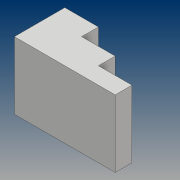
# Autodesk Inventor part: 46 (44000.000 mm^3)
Saved by Autodesk Inventor 2018 (Build 220112000, 112)
## iProperties
Created: 2020-09-18
Part Number: 46 (44000.000 mm^3)
Material: 一般
Document SubType Name: Modeling
Designer: 88697
Density: 1 g/cm^3
Appearance: 預設
Author: 88697
Autodesk Inventor part; units mm, degrees
ref_plane "YZ Plane" through (0, 0, 0) normal (1, 0, 0) x (0, 1, 0)
ref_plane "XZ Plane" through (0, 0, 0) normal (0, 1, 0) x (-1, 0, 0)
ref_plane "XY Plane" through (0, 0, 0) normal (0, 0, 1) x (1, 0, 0)
sketch "草圖1" plane through (0, 0, 0) normal (0, 0, 1) x (1, 0, 0)
  line L0 (0, 0) -> (20, 0)
  line L1 (20, 0) -> (20, 30)
  line L2 (20, 30) -> (0, 30)
  line L3 (0, 30) -> (0, 0)
  line L4 (20, 0) -> (40, 0)
  line L5 (40, 0) -> (40, 20)
  line L6 (40, 20) -> (20, 20)
  line L7 (20, 20) -> (20, 0)
  line L8 (40, 0) -> (60, 0)
  line L9 (60, 0) -> (60, 10)
  line L10 (60, 10) -> (40, 10)
  line L11 (40, 10) -> (40, 0)
  dimension "d0" = 60
  dimension "d1" = 20
  dimension "d2" = 20
  dimension "d3" = 10
  dimension "d4" = 20
  dimension "d5" = 30
  constraints: 24 end point, 6 parallel, 3 horizontal, 3 perpendicular
  measures "d0" distance between parallel lines of L3 L9
  measures "d1" distance of L1.end L2.end
  measures "d2" distance of L9.end L10.end
  measures "d3" distance of L8.end L9.end
  measures "d4" distance of L4.end L5.end
  measures "d5" distance of L0.end L1.end
extrude "擠出1" add sketch "草圖1" along normal blind 40
sketch "草圖2" plane through (20, 20, 0) normal (0, 1, 0) x (1, 0, 0)
  line L0 (0, -30) -> (20, -30)
  line L1 (20, -30) -> (20, -10)
  line L2 (20, -10) -> (0, -10)
  line L3 (0, -10) -> (0, -30)
  line L4 (20, 0) -> (20, -40) projected
  line L5 (20, 0) -> (0, 0) projected
  line L6 (20, -40) -> (0, -40) projected
  line L7 (0, 0) -> (0, -40) projected
  point P0 (-20, 0)
  dimension "d8" = 0
  dimension "d9" = 10
  dimension "d10" = 10
  dimension "d13" = 0
  constraints: 8 end point, 2 parallel, 1 horizontal, 1 perpendicular
  measures "d8" distance between parallel lines of L4 L1
  measures "d9" distance between parallel lines of L5 L2
  measures "d10" distance between parallel lines of L6 L0
  measures "d13" distance between parallel lines of L7 L3
extrude "擠出2" cut sketch "草圖2" against normal up to surface (10 mm away) contours L3 L2 L1 L0
